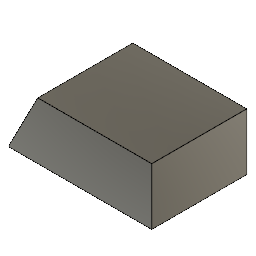
bear_moire (Autodesk Fusion 360 design; units mm, degrees)
Autodesk Fusion 360 part; units mm, degrees
sketch "Sketch1" plane through (0, 0, 0) normal (0, 1, 0) x (1, 0, 0)
  line L0 (0, 0) -> (-75, 0)
  line L1 (-75, -1) -> (-60, -30)
  line L2 (0, -30) -> (0, 0)
  line L3 (-75, 0) -> (-75, -1)
  line L4 (-60, -30) -> (0, -30)
  dimension "d6" = 75
  dimension "d7" = 1
  dimension "d8" = 30
  dimension "d9" = 60
  constraint coincident L0.start L2.end
  constraint horizontal L0
  constraint perpendicular L0 L2
  constraint perpendicular L0 L3
  constraint perpendicular L2 L4
  measures "d6" distance of L0.start L0.end
  measures "d7" distance of L1.start L0.end
  measures "d8" distance of L0 L4
  measures "d9" distance of L1.end L2.start
extrude "Extrude1" add sketch "Sketch1" along normal blind 50
equation "d2 = 50 mm"
equation "d6 = d2 * 1.5"
equation "d7 = ( 0.2 * 5 ) * 1 mm"
